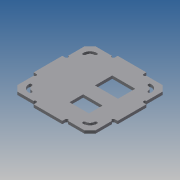
# Autodesk Inventor part: Tapa Enchufes b
Saved by Autodesk Inventor 2017 (Build 210142000, 142)
## iProperties
Part Number: Tapa Enchufes b
Material: Genérico
Document SubType Name: Modeling
Designer: Leo
Density: 1 g/cm^3
Appearance: Valor por defecto
Description: Aluminio compuesto routeado CNC
Author: Leo
Autodesk Inventor part; units mm, degrees
ref_plane "YZ Plane" through (0, 0, 0) normal (1, 0, 0) x (0, 1, 0)
ref_plane "XZ Plane" through (0, 0, 0) normal (0, 1, 0) x (-1, 0, 0)
ref_plane "XY Plane" through (0, 0, 0) normal (0, 0, 1) x (1, 0, 0)
sketch "Boceto1" plane through (0, 0, 0) normal (0, 0, 1) x (1, 0, 0)
  line L0 (-58.5, 20) -> (-58.5, -20)
  line L1 (-58.5, -20) -> (-54.5, -20)
  arc A0 (-54.5, -24) -> (-54.5, -20) centre (-54.5, -22) ccw
  line L2 (-54.5, -24) -> (-54.5, -46.5)
  line L3 (-54.5, -46.5) -> (-46.5, -54.5)
  line L4 (-46.5, -54.5) -> (-24, -54.5)
  arc A1 (-20, -54.5) -> (-24, -54.5) centre (-22, -54.5) ccw
  line L5 (-20, -54.5) -> (-20, -58.5)
  line L6 (-20, -58.5) -> (20, -58.5)
  line L7 (20, -58.5) -> (20, -54.5)
  arc A2 (24, -54.5) -> (20, -54.5) centre (22, -54.5) ccw
  line L8 (24, -54.5) -> (46.5, -54.5)
  line L9 (46.5, -54.5) -> (54.5, -46.5)
  line L10 (27.1297, 0) -> (-27.1297, 0) construction
  line L11 (0, -24.7936) -> (0, 24.7936) construction
  arc A3 (-54.5, 20) -> (-54.5, 24) centre (-54.5, 22) ccw
  line L12 (-54.5, 24) -> (-54.5, 46.5)
  line L13 (-54.5, 46.5) -> (-46.5, 54.5)
  line L14 (-46.5, 54.5) -> (-24, 54.5)
  arc A4 (-24, 54.5) -> (-20, 54.5) centre (-22, 54.5) ccw
  line L15 (-20, 54.5) -> (-20, 58.5)
  line L16 (-20, 58.5) -> (20, 58.5)
  line L17 (20, 58.5) -> (20, 54.5)
  arc A5 (20, 54.5) -> (24, 54.5) centre (22, 54.5) ccw
  line L18 (24, 54.5) -> (46.5, 54.5)
  line L19 (46.5, 54.5) -> (54.5, 46.5)
  line L20 (-54.5, 20) -> (-58.5, 20)
  line L21 (58.5, 20) -> (58.5, -20)
  line L22 (58.5, -20) -> (54.5, -20)
  arc A6 (54.5, -20) -> (54.5, -24) centre (54.5, -22) ccw
  line L23 (54.5, -24) -> (54.5, -46.5)
  line L24 (54.5, 24) -> (54.5, 46.5)
  arc A7 (54.5, 24) -> (54.5, 20) centre (54.5, 22) ccw
  line L25 (54.5, 20) -> (58.5, 20)
  line L26 (32, 7) -> (32, 31)
  line L27 (32, 31) -> (0, 31)
  line L28 (0, 31) -> (0, 7)
  line L29 (0, 7) -> (32, 7)
  line L30 (-19.5, 34.5) -> (-19.5, 3.5) construction
  line L31 (-19.5, 3.5) -> (51.5, 3.5) construction
  line L32 (51.5, 3.5) -> (51.5, 34.5) construction
  line L33 (51.5, 34.5) -> (-19.5, 34.5) construction
  line L34 (29.5, -12) -> (2.5, -12)
  line L35 (2.5, -12) -> (2.5, -31)
  line L36 (2.5, -31) -> (29.5, -31)
  line L37 (29.5, -31) -> (29.5, -12)
  arc A8 (37.5, -45.5) -> (45.5, -37.5) centre (37.5, -37.5) ccw construction
  arc A9 (37.5, -47.6) -> (47.6, -37.5) centre (37.5, -37.5) ccw
  arc A10 (37.5, -43.4) -> (43.4, -37.5) centre (37.5, -37.5) ccw
  arc A11 (37.5, -43.4) -> (37.5, -47.6) centre (37.5, -45.5) ccw
  arc A12 (47.6, -37.5) -> (43.4, -37.5) centre (45.5, -37.5) ccw
  arc A13 (47.6, 37.5) -> (37.5, 47.6) centre (37.5, 37.5) ccw
  arc A14 (43.4, 37.5) -> (37.5, 43.4) centre (37.5, 37.5) ccw
  arc A15 (37.5, 47.6) -> (37.5, 43.4) centre (37.5, 45.5) ccw
  arc A16 (43.4, 37.5) -> (47.6, 37.5) centre (45.5, 37.5) ccw
  arc A17 (-47.6, -37.5) -> (-37.5, -47.6) centre (-37.5, -37.5) ccw
  arc A18 (-43.4, -37.5) -> (-37.5, -43.4) centre (-37.5, -37.5) ccw
  arc A19 (-37.5, -47.6) -> (-37.5, -43.4) centre (-37.5, -45.5) ccw
  arc A20 (-43.4, -37.5) -> (-47.6, -37.5) centre (-45.5, -37.5) ccw
  arc A21 (-37.5, 43.4) -> (-43.4, 37.5) centre (-37.5, 37.5) ccw
  arc A22 (-47.6, 37.5) -> (-43.4, 37.5) centre (-45.5, 37.5) ccw
  arc A23 (-37.5, 47.6) -> (-47.6, 37.5) centre (-37.5, 37.5) ccw
  arc A24 (-37.5, 43.4) -> (-37.5, 47.6) centre (-37.5, 45.5) ccw
  point P0 (0, 0)
  point P1 (0, 0)
  point P2 (-58.5, 0)
  point P3 (0, 58.5)
  point P4 (16, 34.5)
  point P5 (16, 31)
  point P6 (51.5, 19)
  point P7 (32, 19)
  point P8 (16, -12)
  point P9 (16, 7)
  dimension "d0" = 40
  dimension "d1" = 4
  dimension "d2" = 2
  dimension "d3" = 109
  dimension "d4" = 117
  dimension "d5" = 4
  dimension "d6" = 8
  dimension "d10" = 24
  dimension "d11" = 32
  dimension "d12" = 31
  dimension "d13" = 71
  dimension "d14" = 3
  dimension "d15" = 20
  dimension "d16" = 19
  dimension "d17" = 27
  dimension "d19" = 24
  dimension "d22" = 2.1
  dimension "d23" = 8
  dimension "d24" = 75
  dimension "d25" = 75
  dimension "d26" = 109
  constraints: 76 end point, 50 point on circle, 46 symmetric about line, 25 centre point, 13 point on line, 11 perpendicular, 10 midpoint, 7 parallel, 7 tangent, 5 horizontal, 3 horizontal alignment, 3 vertical alignment, 2 equal radius, 2 vertical, 1 coincident, 17 other
  measures "d0" distance of L0.start L0.end
  measures "d1" distance between parallel lines of L2 L0
  measures "d2" radius of A3
  measures "d3" distance between parallel lines of L24 L12
  measures "d4" distance between parallel lines of L6 L16
  measures "d5" distance between parallel lines of L16 L18
  measures "d6" horizontal distance of L8.end L9.end
  measures "d10" distance of L26.start L26.end
  measures "d11" distance of L26.end L27.end
  measures "d12" distance of L30.start L30.end
  measures "d13" distance of L30.end L31.end
  measures "d14" distance between parallel lines of L24 L32
  measures "d15" distance between parallel lines of L18 L33
  measures "d16" distance of L34.end L35.end
  measures "d17" distance of L34.start L34.end
  measures "d19" diameter of L34 L10
  measures "d22" radius of A12
  measures "d23" distance of A8.end A8.centre
  measures "d24" distance of A18.centre A8.centre
  measures "d25" distance of A14.centre A8.centre
  measures "d26" distance between parallel lines of L8 L18
extrude "Extrusión1" add sketch "Boceto1" along normal blind 4
equation "\"d5\" = d1"
equation "\"d25\" = d24"
